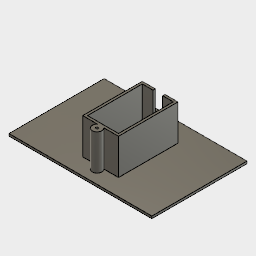
motor_mount (Autodesk Fusion 360 design; units mm, degrees)
Autodesk Fusion 360 part; units mm, degrees
sketch "Sketch1" plane through (0, 0, 0) normal (0, 1, 0) x (1, 0, 0)
  line L0 (0, 0) -> (0, -40)
  line L1 (0, -40) -> (60, -40)
  line L2 (60, -40) -> (60, 0)
  line L3 (60, 0) -> (0, 0)
  dimension "d1" = 60
  dimension "d2" = 40
  dimension "d3" = 90
  dimension "d4" = 90
  measures "d1" distance of L0.end L1.end
  measures "d2" distance of L0.start L0.end
  measures "d3" angle of L2 L3
  measures "d4" angle of L0 L3
extrude "Extrude1" add sketch "Sketch1" along normal blind 1
sketch "Sketch2" plane through (0, 1, 0) normal (0, 1, 0) x (-1, 0, 0)
  line L0 (-60, 0) -> (0, 0)
  line L1 (0, 0) -> (0, 40)
  line L2 (0, 40) -> (-60, 40)
  line L3 (-60, 40) -> (-60, 0)
  line L4 (-24, 8) -> (-39, 8)
  line L5 (-39, 8) -> (-39, 33)
  line L6 (-39, 33) -> (-24, 33)
  line L7 (-24, 33) -> (-24, 8)
  dimension "d18" = 15
  dimension "d19" = 25
  dimension "d20" = 24
  dimension "d21" = 8
  measures "d18" distance of L4.start L4.end
  measures "d19" distance of L4.start L6.end
  measures "d20" distance of L1 L7
  measures "d21" distance of L0 L4
extrude "Extrude2" add sketch "Sketch2" along normal blind 10 contours L4 L5 L6 L7
sketch "Sketch3" plane through (0, 11, 0) normal (0, 1, 0) x (-1, 0, 0)
  line L0 (-24, 33) -> (-39, 33)
  line L1 (-39, 33) -> (-39, 8)
  line L2 (-39, 8) -> (-24, 8)
  line L3 (-24, 8) -> (-24, 33)
  line L4 (-25, 9) -> (-38, 9)
  line L5 (-38, 9) -> (-38, 32)
  line L6 (-38, 32) -> (-25, 32)
  line L7 (-25, 32) -> (-25, 9)
  line L8 (-29.5, 8) -> (-29.5, 9)
  line L9 (-33.5, 8) -> (-33.5, 9)
  dimension "d24" = 1
  dimension "d25" = 1
  dimension "d26" = 1
  dimension "d27" = 1
  dimension "d28" = 4
  dimension "d29" = 5.5
  measures "d24" distance of L3 L7
  measures "d25" distance of L1 L5
  measures "d26" distance of L2 L4
  measures "d27" distance of L0 L6
  measures "d28" distance of L8.end L9.end
  measures "d29" distance of L2.end L8.start
extrude "Extrude3" cut sketch "Sketch3" against normal blind 10 contours L2 L4 L8 L9 | L4 L5 L6 L7
sketch "Sketch4" plane through (0, 1, 0) normal (0, 1, 0) x (-1, 0, 0)
  line L0 (-24, 33) -> (-24, 8)
  line L1 (-24, 8) -> (-29.5, 8)
  line L2 (-29.5, 8) -> (-29.5, 9)
  line L3 (-29.5, 9) -> (-25, 9)
  line L4 (-25, 9) -> (-25, 32)
  line L5 (-25, 32) -> (-38, 32)
  line L6 (-38, 32) -> (-38, 9)
  line L7 (-38, 9) -> (-33.5, 9)
  line L8 (-33.5, 9) -> (-33.5, 8)
  line L9 (-33.5, 8) -> (-39, 8)
  line L10 (-39, 8) -> (-39, 33)
  line L11 (-39, 33) -> (-24, 33)
  line L12 (-60, 0) -> (0, 0)
  line L13 (0, 0) -> (0, 40)
  line L14 (0, 40) -> (-60, 40)
  line L15 (-60, 40) -> (-60, 0)
  circle A0 centre (-31.5, 34.5) radius 2
  circle A1 centre (-31.5, 34.5) radius 0.5
  dimension "d32" = 1
  dimension "d33" = 4
  dimension "d35" = 2.5
  dimension "d36" = 6.5
  measures "d32" diameter of A1
  measures "d33" diameter of A0
  measures "d35" distance of L5 A0.centre
  measures "d36" distance of L6 A0.centre
extrude "Extrude4" add sketch "Sketch4" along normal blind 15 contours L11 A0 picked at (-31.4875, 33.3338)
sketch "Sketch5" plane through (0, 0, 0) normal (0, 0, 1) x (1, 0, 0)
extrude "Extrude5" add 1 faces at (31.4875, 16, 33.3338) along direction (0, -1, 0) blind 5
extrude "Extrude6" add 1 faces at (31.059, 11, 32.3333) along direction (0, 1, 0) blind 5
named bodies: "motor_stand"
